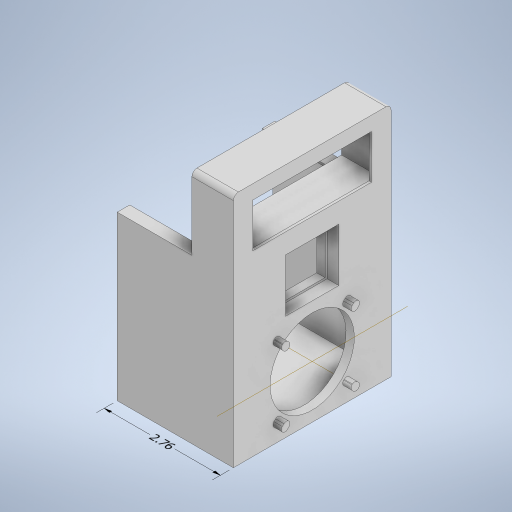
# Autodesk Inventor part: PICHero Case
Saved by Autodesk Inventor 2024 (Build 280153000, 153)
## iProperties
Created: 2023-04-17
Part Number: PICHero Case
Material: Generic
Document SubType Name: Modeling
Designer: artis
Density: 1 g/cm^3
Appearance: Default
Author: artis
## iProperties of the stored document InterfaceCase_3DPrint.ipt
Created: 2023-04-17
Part Number: InterfaceCase_3DPrint
Material: Generic
Document SubType Name: Modeling
Designer: artis
Density: 1 g/cm^3
Appearance: Default
Author: artis
Autodesk Inventor part; units mm, degrees
ref_plane "YZ Plane" through (0, 0, 0) normal (1, 0, 0) x (0, 1, 0)
ref_plane "XZ Plane" through (0, 0, 0) normal (0, 1, 0) x (-1, 0, 0)
ref_plane "XY Plane" through (0, 0, 0) normal (0, 0, 1) x (1, 0, 0)
sketch "Sketch1" plane through (0, 0, 0) normal (1, 0, 0) x (0, 1, 0)
  line L0 (-26.3, 26.3) -> (26.3, 26.3)
  line L1 (26.3, 26.3) -> (26.3, -26.3)
  line L2 (26.3, -26.3) -> (-26.3, -26.3)
  line L3 (-26.3, -26.3) -> (-26.3, 26.3)
  line L4 (63.625, 16) -> (31.625, 16)
  line L5 (31.625, 16) -> (31.625, -16)
  line L6 (31.625, -16) -> (63.625, -16)
  line L7 (63.625, -16) -> (63.625, 16)
  circle A0 centre (0, 0) radius 25.4
  line L8 (0, -31.75) -> (21, -31.75) construction
  line L9 (0, 31.75) -> (21, 31.75) construction
  line L10 (21, 31.75) -> (21, -31.75) construction
  line L11 (-26.3, 26.3) -> (26.3, -26.3) construction
  line L12 (22.0607, -18.9494) -> (23.0506, -19.9393)
  line L13 (23.0506, -22.7678) -> (22.7678, -23.0506)
  line L14 (19.9393, -23.0506) -> (18.9494, -22.0607)
  line L15 (18.9494, -19.2322) -> (19.2322, -18.9494)
  line L16 (20.6464, -17.5352) -> (21.3536, -24.4648) construction
  line L17 (24.4648, -21.3536) -> (17.5352, -20.6464) construction
  arc A1 (23.0506, -22.7678) -> (23.0506, -19.9393) centre (21.6364, -21.3536) ccw
  arc A2 (19.9393, -23.0506) -> (22.7678, -23.0506) centre (21.3536, -21.6364) ccw
  arc A3 (18.9494, -19.2322) -> (18.9494, -22.0607) centre (20.3636, -20.6464) ccw
  arc A4 (22.0607, -18.9494) -> (19.2322, -18.9494) centre (20.6464, -20.3636) ccw
  line L18 (18.9494, 22.0607) -> (19.9393, 23.0506)
  arc A5 (22.7678, 23.0506) -> (19.9393, 23.0506) centre (21.3536, 21.6364) ccw
  arc A6 (18.9494, 22.0607) -> (18.9494, 19.2322) centre (20.3636, 20.6464) ccw
  line L19 (23.0506, 19.9393) -> (22.0607, 18.9494)
  arc A7 (19.2322, 18.9494) -> (22.0607, 18.9494) centre (20.6464, 20.3636) ccw
  arc A8 (23.0506, 19.9393) -> (23.0506, 22.7678) centre (21.6364, 21.3536) ccw
  line L20 (22.7678, 23.0506) -> (23.0506, 22.7678)
  line L21 (19.2322, 18.9494) -> (18.9494, 19.2322)
  line L22 (-22.0607, 18.9494) -> (-23.0506, 19.9393)
  arc A9 (-23.0506, 22.7678) -> (-23.0506, 19.9393) centre (-21.6364, 21.3536) ccw
  arc A10 (-22.0607, 18.9494) -> (-19.2322, 18.9494) centre (-20.6464, 20.3636) ccw
  line L23 (-19.9393, 23.0506) -> (-18.9494, 22.0607)
  arc A11 (-18.9494, 19.2322) -> (-18.9494, 22.0607) centre (-20.3636, 20.6464) ccw
  arc A12 (-19.9393, 23.0506) -> (-22.7678, 23.0506) centre (-21.3536, 21.6364) ccw
  line L24 (-23.0506, 22.7678) -> (-22.7678, 23.0506)
  line L25 (-18.9494, 19.2322) -> (-19.2322, 18.9494)
  line L26 (-18.9494, -22.0607) -> (-19.9393, -23.0506)
  arc A13 (-22.7678, -23.0506) -> (-19.9393, -23.0506) centre (-21.3536, -21.6364) ccw
  arc A14 (-18.9494, -22.0607) -> (-18.9494, -19.2322) centre (-20.3636, -20.6464) ccw
  line L27 (-23.0506, -19.9393) -> (-22.0607, -18.9494)
  arc A15 (-19.2322, -18.9494) -> (-22.0607, -18.9494) centre (-20.6464, -20.3636) ccw
  arc A16 (-23.0506, -19.9393) -> (-23.0506, -22.7678) centre (-21.6364, -21.3536) ccw
  line L28 (-22.7678, -23.0506) -> (-23.0506, -22.7678)
  line L29 (-19.2322, -18.9494) -> (-18.9494, -19.2322)
  line L30 (66.675, 42.5) -> (66.675, 47.5)
  line L31 (102.15, -35.75) -> (75.65, -35.75)
  line L32 (75.65, -35.75) -> (75.65, 35.75)
  line L33 (75.65, 35.75) -> (102.15, 35.75)
  line L34 (102.15, 35.75) -> (102.15, -35.75)
  line L35 (102.15, -35.75) -> (75.65, 35.75) construction
  line L36 (75.65, -35.75) -> (102.15, 35.75) construction
  line L37 (66.675, 47.5) -> (-31.75, 47.5)
  line L38 (66.675, 42.5) -> (66.675, 0)
  line L39 (66.675, 0) -> (66.675, -47.5)
  line L40 (-31.75, 47.5) -> (-31.75, -47.5)
  line L41 (-31.75, -47.5) -> (66.675, -47.5)
  line L42 (66.675, 47.5) -> (110.675, 47.5)
  line L43 (110.675, 47.5) -> (110.675, -47.5)
  line L44 (110.675, -47.5) -> (66.675, -47.5)
  point P0 (47.625, 0)
  point P1 (21, -21)
  point P2 (21, 21)
  point P3 (21.3536, 24.4648)
  point P4 (17.5352, 20.6464)
  point P5 (24.4648, 21.3536)
  point P6 (20.6464, 17.5352)
  point P7 (-21, 21)
  point P8 (-24.4648, 21.3536)
  point P9 (-20.6464, 17.5352)
  point P10 (-21.3536, 24.4648)
  point P11 (-17.5352, 20.6464)
  point P12 (-21, -21)
  point P13 (-21.3536, -24.4648)
  point P14 (-17.5352, -20.6464)
  point P15 (-24.4648, -21.3536)
  point P16 (-20.6464, -17.5352)
  point P17 (88.9, 0)
  dimension "d0" = 52.6
  dimension "d1" = 52.6
  dimension "d2" = 32
  dimension "d3" = 32
  dimension "d4" = 50.8
  dimension "d5" = 21
  dimension "d6" = 21
  dimension "d7" = 5.4
  dimension "d8" = 4.4
  dimension "d9" = 2
  dimension "d12" = 360
  dimension "d15" = 5
  dimension "d16" = 71.5
  dimension "d17" = 26.5
  dimension "d18" = 47.5
  dimension "d19" = 47.5
  dimension "d20" = 44
  dimension "d21" = 95
  constraints: 90 end point, 35 point on line, 32 point on circle, 17 centre point, 10 parallel, 8 tangent, 6 horizontal, 6 perpendicular, 4 midpoint, 3 equal radius, 3 vertical, 1 coincident, 1 collinear, 101 other
  measures "d0" distance of L1.end L2.end
  measures "d1" distance of L0.end L1.end
  measures "d2" distance of L6.end L5.end
  measures "d3" distance of L5.end L4.end
  measures "d4" diameter of A0
  measures "d5" distance of L8.start L8.end
  measures "d6" distance of L9.start L9.end
  measures "d7" distance of L16.start L17.start
  measures "d8" distance of L17.start L16.end
  measures "d9" radius of A1
  measures "d15" distance of L30.start L30.end
  measures "d16" distance of L31.end L32.end
  measures "d17" distance of L31.start L31.end
  measures "d18" distance of L38.end L30.end
  measures "d19" distance of L38.end L39.end
  measures "d20" distance of L30.end L42.end
  measures "d21" distance of L42.end L43.end
extrude "Extrusion1" add sketch "Sketch1" against normal blind 70 contours L0 L1 L2 L3 | L38 L39 L41 L40 L37 L30
extrude "Extrusion2" add sketch "Sketch1" along normal blind 5 contours L12 A1 L13 A2 L14 A3 L15 A4 | L18 A5 L20 A8 L19 A7 L21 A6 | L22 A9 L24 A12 L23 A11 L25 A10 | L26 A13 L28 A16 L27 A15 L29 A14
sketch "Sketch2" plane through (0, 0, 0) normal (1, 0, 0) x (0, 1, 0)
  line L0 (103.9, 42.75) -> (73.9, 42.75)
  line L1 (73.9, 42.75) -> (73.9, -42.75)
  line L2 (73.9, -42.75) -> (103.9, -42.75)
  line L3 (103.9, -42.75) -> (103.9, 42.75)
  line L4 (103.9, 42.75) -> (73.9, -42.75) construction
  line L5 (73.9, 42.75) -> (103.9, -42.75) construction
  point P0 (0, 0)
  point P1 (88.9, 0)
  dimension "d27" = 85.5
  dimension "d28" = 30
  constraints: 12 end point, 2 midpoint, 2 parallel, 1 horizontal, 1 perpendicular
  measures "d27" distance of L1.end L0.end
  measures "d28" distance of L1.end L2.end
extrude "Extrusion4" add sketch "Sketch2" against normal blind 1.5
extrude "Extrusion5" cut sketch "Sketch1" against normal blind 1.5 contours L31 L32 L33 L34
sketch "Sketch3" plane through (0, 0, 0) normal (1, 0, 0) x (0, 1, 0)
  line L0 (103.9, 42.75) -> (73.9, 42.75) projected
  line L1 (103.9, 42.75) -> (73.9, 42.75)
  line L2 (73.9, 42.75) -> (73.9, -42.75)
  line L3 (73.9, -42.75) -> (103.9, -42.75)
  line L4 (103.9, -42.75) -> (103.9, 42.75)
  line L5 (66.675, 47.5) -> (110.675, 47.5) projected
  line L6 (110.675, 47.5) -> (110.675, -47.5) projected
  line L7 (66.675, -47.5) -> (66.675, 47.5) projected
  line L8 (110.675, 47.5) -> (66.675, 47.5)
  line L9 (66.675, 47.5) -> (66.675, -47.5)
  line L10 (66.675, -47.5) -> (110.675, -47.5)
  line L11 (110.675, -47.5) -> (110.675, 47.5)
  point P0 (0, 0)
  constraints: 16 end point, 4 parallel, 2 horizontal, 2 perpendicular
extrude "Extrusion6" add sketch "Sketch3" against normal blind 25
shell "Shell2" thickness 1.25 removed faces 1 at (-70, 12.6622, 40.0716)
sketch "Sketch4" plane through (-70, 0, 0) normal (-1, 0, 0) x (0, 0, 1)
  arc A0 (17.1213, 20.4226) -> (-17.1213, 20.4226) centre (0, 0) ccw projected
  arc A1 (23.6517, 23.9345) -> (19.0555, 23.9345) centre (21.3536, 21.6364) ccw projected
  arc A2 (23.9345, 19.0555) -> (23.9345, 23.6517) centre (21.6364, 21.3536) ccw projected
  arc A3 (23.0506, 19.9393) -> (23.0506, 22.7678) centre (21.6364, 21.3536) ccw projected
  line L0 (46.25, -30.5) -> (-46.25, -30.5) projected
  line L1 (46.25, 109.425) -> (46.25, -30.5) projected
  line L2 (-46.25, 109.425) -> (46.25, 109.425) projected
  line L3 (-46.25, -30.5) -> (-46.25, 109.425) projected
  line L4 (17.25, 64.875) -> (-17.25, 64.875) projected
  line L5 (17.25, 30.375) -> (17.25, 64.875) projected
  line L6 (-17.25, 30.375) -> (17.25, 30.375) projected
  line L7 (-17.25, 64.875) -> (-17.25, 30.375) projected
  arc A4 (-22.9445, 18.0655) -> (-20.4226, 17.1213) centre (-20.6464, 20.3636) ccw projected
  line L8 (-23.9345, 19.0555) -> (-22.9445, 18.0655) projected
  arc A5 (-23.9345, 23.6517) -> (-23.9345, 19.0555) centre (-21.6364, 21.3536) ccw projected
  line L9 (-23.6517, 23.9345) -> (-23.9345, 23.6517) projected
  arc A6 (-19.0555, 23.9345) -> (-23.6517, 23.9345) centre (-21.3536, 21.6364) ccw projected
  line L10 (-18.0655, 22.9445) -> (-19.0555, 23.9345) projected
  arc A7 (-17.1213, 20.4226) -> (-18.0655, 22.9445) centre (-20.3636, 20.6464) ccw projected
  arc A8 (17.1213, 20.4226) -> (-17.1213, 20.4226) centre (0, 0) ccw projected
  arc A9 (18.0655, 22.9445) -> (17.1213, 20.4226) centre (20.3636, 20.6464) ccw projected
  line L11 (19.0555, 23.9345) -> (18.0655, 22.9445) projected
  arc A10 (23.6517, 23.9345) -> (19.0555, 23.9345) centre (21.3536, 21.6364) ccw projected
  line L12 (23.9345, 23.6517) -> (23.6517, 23.9345) projected
  arc A11 (23.9345, 19.0555) -> (23.9345, 23.6517) centre (21.6364, 21.3536) ccw projected
  line L13 (22.9445, 18.0655) -> (23.9345, 19.0555) projected
  arc A12 (20.4226, 17.1213) -> (22.9445, 18.0655) centre (20.6464, 20.3636) ccw projected
  arc A13 (20.4226, -17.1213) -> (20.4226, 17.1213) centre (0, 0) ccw projected
  arc A14 (22.9445, -18.0655) -> (20.4226, -17.1213) centre (20.6464, -20.3636) ccw projected
  line L14 (23.9345, -19.0555) -> (22.9445, -18.0655) projected
  arc A15 (23.9345, -23.6517) -> (23.9345, -19.0555) centre (21.6364, -21.3536) ccw projected
  line L15 (23.6517, -23.9345) -> (23.9345, -23.6517) projected
  arc A16 (19.0555, -23.9345) -> (23.6517, -23.9345) centre (21.3536, -21.6364) ccw projected
  line L16 (18.0655, -22.9445) -> (19.0555, -23.9345) projected
  arc A17 (17.1213, -20.4226) -> (18.0655, -22.9445) centre (20.3636, -20.6464) ccw projected
  arc A18 (-17.1213, -20.4226) -> (17.1213, -20.4226) centre (0, 0) ccw projected
  arc A19 (-18.0655, -22.9445) -> (-17.1213, -20.4226) centre (-20.3636, -20.6464) ccw projected
  line L17 (-19.0555, -23.9345) -> (-18.0655, -22.9445) projected
  arc A20 (-23.6517, -23.9345) -> (-19.0555, -23.9345) centre (-21.3536, -21.6364) ccw projected
  line L18 (-23.9345, -23.6517) -> (-23.6517, -23.9345) projected
  arc A21 (-23.9345, -19.0555) -> (-23.9345, -23.6517) centre (-21.6364, -21.3536) ccw projected
  line L19 (-22.9445, -18.0655) -> (-23.9345, -19.0555) projected
  arc A22 (-20.4226, -17.1213) -> (-22.9445, -18.0655) centre (-20.6464, -20.3636) ccw projected
  arc A23 (-20.4226, 17.1213) -> (-20.4226, -17.1213) centre (0, 0) ccw projected
  line L20 (44, 105.15) -> (44, 72.65) projected
  line L21 (44, 72.65) -> (-44, 72.65) projected
  line L22 (-44, 72.65) -> (-44, 105.15) projected
  line L23 (-44, 105.15) -> (44, 105.15) projected
  point P0 (22.7678, 23.0506)
  point P1 (19.0555, 23.9345)
extrude "Extrusion7" cut sketch "Sketch4" against normal blind 65 contours A9 L11 A1 L12 A2 L13 A12 A13 A14 L14 A15 L15 A16 L16 A17 A18 A19 L17 A20 L18 A21 L19 A22 A23 A4 L8 A5 L9 A6 L10 A7 A0
sketch "Sketch5" plane through (-70, 0, 0) normal (-1, 0, 0) x (0, 0, 1)
  line L0 (17.25, 64.875) -> (-17.25, 64.875) projected
  line L1 (-16, 63.625) -> (16, 63.625) projected
  line L2 (-17.25, 64.875) -> (-17.25, 30.375) projected
  line L3 (-16, 31.625) -> (-16, 63.625) projected
  line L4 (16, 31.625) -> (-16, 31.625) projected
  line L5 (-17.25, 30.375) -> (17.25, 30.375) projected
  line L6 (16, 63.625) -> (16, 31.625) projected
  line L7 (17.25, 30.375) -> (17.25, 64.875) projected
  point P0 (0, 0)
extrude "Extrusion8" cut sketch "Sketch5" against normal blind 63 contours L7 L5 L2 L0 | L1 L6 L4 L3
sketch "Sketch6" plane through (-7, 0, 0) normal (-1, 0, 0) x (0, 0, 1)
  line L0 (-16, 63.625) -> (-16, 31.625) projected
  line L1 (16, 63.625) -> (-16, 63.625) projected
  line L2 (16, 31.625) -> (16, 63.625) projected
  line L3 (-16, 31.625) -> (16, 31.625) projected
  line L4 (-17.25, 30.375) -> (-17.25, 64.875) projected
  line L5 (17.25, 30.375) -> (-17.25, 30.375) projected
  line L6 (17.25, 64.875) -> (17.25, 30.375) projected
  line L7 (-17.25, 64.875) -> (17.25, 64.875) projected
  line L8 (-16, 31.625) -> (16, 31.625) projected
  line L9 (-14.75, 50.8) -> (-14.75, 32.875)
  line L10 (-14.75, 50.8) -> (3.175, 50.8) construction
  line L11 (-14.75, 32.875) -> (0, 32.875)
  line L12 (-14.75, 63.625) -> (-14.75, 62.375) construction
  line L13 (-14.75, 62.375) -> (-14.75, 50.8)
  line L14 (0, 62.375) -> (-14.75, 62.375)
  line L15 (14.75, 50.8) -> (14.75, 32.875)
  line L16 (14.75, 32.875) -> (0, 32.875)
  line L17 (14.75, 62.375) -> (14.75, 50.8)
  line L18 (0, 62.375) -> (14.75, 62.375)
  point P0 (0, 0)
  dimension "d50" = 90
  dimension "d51" = 1.25
  constraints: 20 end point, 3 perpendicular, 1 horizontal, 1 point on line, 1 vertical
  measures "d50" angle of L9 L10
  measures "d51" distance of L12.start L12.end
extrude "Extrusion9" add sketch "Sketch6" along normal blind 5 contours L1 L2 L3 L0 | L4 L7 L6 L5
sketch "Sketch7" plane through (-70, 66.675, 47.5) normal (0, 1, 0) x (1, 0, 0)
  line L0 (45, 0) -> (45, 95) projected
  line L1 (5.8, 87.5) -> (45, 87.5)
  line L2 (45, 87.5) -> (45, 7.5)
  line L3 (45, 7.5) -> (5.8, 7.5)
  line L4 (5.8, 87.5) -> (45, 7.5) construction
  line L5 (45, 87.5) -> (5.8, 7.5) construction
  line L6 (0, 95) -> (0, 0) projected
  line L7 (5.8, 87.5) -> (0, 87.5)
  line L8 (0, 87.5) -> (0, 7.5)
  line L9 (0, 7.5) -> (5.8, 7.5)
  point P0 (70, 47.5)
  point P1 (25.4, 47.5)
  dimension "d54" = 80
  constraints: 16 end point, 2 horizontal, 2 midpoint, 2 parallel, 2 perpendicular, 2 point on line
  measures "d54" distance of L1.end L2.end
extrude "Extrusion10" cut sketch "Sketch7" against normal blind 5
fillet "Fillet1" radius 3 2 edges at (-12.5, 110.675, -47.5) (-12.5, 110.675, 47.5)
body "Solid1"
